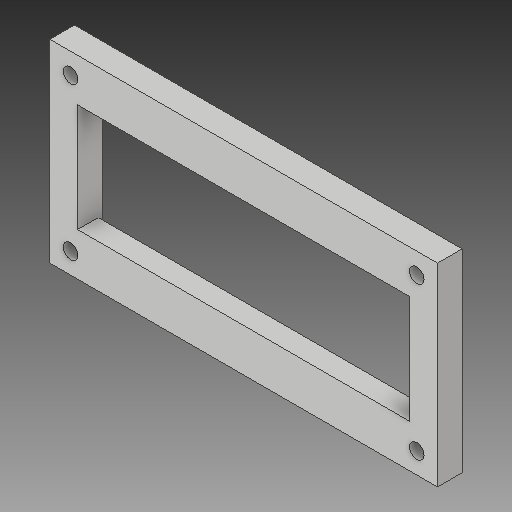
# Autodesk Inventor part: RampPanell
Saved by Autodesk Inventor 2018 (Build 220112000, 112)
## iProperties
Created: 2020-03-31
Part Number: RampPanell
Material: Generic
Document SubType Name: Modeling
Designer: emile
Density: 1 g/cm^3
Appearance: Default
Mass: 89.9991 g
Surface Area: 278.054 cm^2
Volume: 89.9991 cm^3
Author: emile
Autodesk Inventor part; units mm, degrees
ref_plane "YZ Plane" through (0, 0, 0) normal (1, 0, 0) x (0, 1, 0)
ref_plane "XZ Plane" through (0, 0, 0) normal (0, 1, 0) x (-1, 0, 0)
ref_plane "XY Plane" through (0, 0, 0) normal (0, 0, 1) x (1, 0, 0)
sketch "Sketch6" plane through (0, 0, 0) normal (0, 0, 1) x (1, 0, 0)
  line L0 (88.9, -44.45) -> (-88.9, -44.45)
  line L1 (-88.9, -44.45) -> (-88.9, 44.45)
  line L2 (-88.9, 44.45) -> (88.9, 44.45)
  line L3 (88.9, 44.45) -> (88.9, -44.45)
  line L4 (88.9, -44.45) -> (-88.9, 44.45) construction
  line L5 (-88.9, -44.45) -> (88.9, 44.45) construction
  line L6 (76.2, -27.94) -> (-76.2, -27.94)
  line L7 (-76.2, -27.94) -> (-76.2, 27.94)
  line L8 (-76.2, 27.94) -> (76.2, 27.94)
  line L9 (76.2, 27.94) -> (76.2, -27.94)
  line L10 (76.2, -27.94) -> (-76.2, 27.94) construction
  line L11 (-76.2, -27.94) -> (76.2, 27.94) construction
  point P0 (0, 0)
  dimension "d36" = 177.8
  dimension "d37" = 88.9
  dimension "d38" = 55.88
  dimension "d39" = 152.4
  constraints: 24 end point, 4 midpoint, 4 parallel, 2 horizontal, 2 perpendicular
  measures "d36" distance of L1.end L2.end
  measures "d37" distance of L2.end L0.start
  measures "d38" distance of L6.end L7.end
  measures "d39" distance of L7.end L8.end
extrude "Extrusion6" add sketch "Sketch6" along normal blind 1.778
sketch "Sketch7" plane through (0, 0, 1.778) normal (0, 0, 1) x (1, 0, 0)
  line L0 (-76.2, -27.94) -> (-76.2, 27.94) projected
  line L1 (-76.2, 27.94) -> (76.2, 27.94) projected
  line L2 (76.2, 27.94) -> (76.2, -27.94) projected
  line L3 (76.2, -27.94) -> (-76.2, -27.94) projected
  line L4 (-88.9, -44.45) -> (88.9, -44.45) projected
  line L5 (88.9, -44.45) -> (88.9, 44.45) projected
  line L6 (88.9, 44.45) -> (-88.9, 44.45) projected
  line L7 (-88.9, 44.45) -> (-88.9, -44.45) projected
  line L8 (-76.2, 27.94) -> (76.2, 27.94)
  line L9 (76.2, 27.94) -> (76.2, 24.765)
  line L10 (76.2, 24.765) -> (-76.2, 24.765)
  line L11 (-76.2, 24.765) -> (-76.2, 27.94)
  line L12 (76.2, -27.94) -> (-76.2, -27.94) projected
  line L13 (-76.2, -27.94) -> (76.2, -27.94)
  line L14 (76.2, -27.94) -> (76.2, -24.765)
  line L15 (76.2, -24.765) -> (-76.2, -24.765)
  line L16 (-76.2, -24.765) -> (-76.2, -27.94)
  point P0 (0, 0)
  dimension "d42" = 3.175
  dimension "d43" = 3.175
  constraints: 16 end point, 4 parallel, 4 perpendicular
  measures "d42" distance between parallel lines of L1 L10
  measures "d43" distance between parallel lines of L3 L15
extrude "Extrusion7" add sketch "Sketch7" along normal blind 9.525 contours L0 L15 L2 L3 | L0 L1 L2 L10 | L7 L6 L5 L4
sketch "Sketch8" plane through (0, 0, 0) normal (0, 0, -1) x (-1, 0, 0)
  point P0 (79.375, -34.925)
  point P1 (-79.375, -34.925)
  point P2 (-79.375, 34.925)
  point P3 (79.375, 34.925)
hole "Hole2" at (-79.375, -34.925, 0) at (79.375, -34.925, 0) at (79.375, 34.925, 0) at (-79.375, 34.925, 0) direction (0, 0, 1) diameter 6.7564 depth 11.303
body "Solid2"
